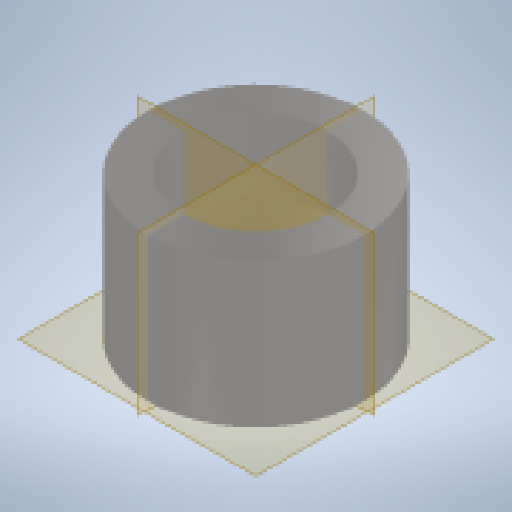
# Autodesk Inventor part: Z0
Saved by Autodesk Inventor 2025.2 (Build 292293000, 293)
## iProperties
Created: 2025-03-22
Part Number: Z0
Material: Steel, Alloy
Document SubType Name: Modeling
Designer: MSIGAMING
Mass: 84995.8 g
Surface Area: 3926.99 cm^2
Volume: 10995.6 cm^3
Density: 7.73 g/cm^3
Appearance: Semi-Polished
Author: MSIGAMING
Autodesk Inventor part; units mm, degrees
sketch "Sketch1" plane through (0, 0, 0) normal (0, 1, 0) x (-1, 0, 0)
  circle A0 centre (0, 0) radius 150
  dimension "d0" = 300
  constraints: 1 centre point, 1 coincident
  measures "d0" diameter of A0
extrude "Extrusion1" add sketch "Sketch1" along normal blind 200
sketch "Sketch2" plane through (0, 200, 0) normal (0, 1, 0) x (1, 0, 0)
  circle A0 centre (0, 0) radius 100
  dimension "d3" = 200
  constraints: 1 centre point, 1 coincident
  measures "d3" diameter of A0
extrude "Extrusion2" cut sketch "Sketch2" against normal blind 100
body "Solid1"
